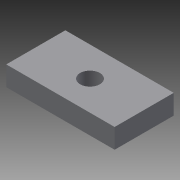
# Autodesk Inventor part: p1-1
Saved by Autodesk Inventor 2014 (Build 180170000, 170)
## iProperties
Created: 2017-02-06
Part Number: p1-1
Material: Generic
Document SubType Name: Modeling
Designer: mschaffel
Density: 1 g/cm^3
Appearance: Default
Author: mschaffel
Autodesk Inventor part; units mm, degrees
ref_plane "YZ Plane" through (0, 0, 0) normal (1, 0, 0) x (0, 1, 0)
ref_plane "XZ Plane" through (0, 0, 0) normal (0, 1, 0) x (-1, 0, 0)
ref_plane "XY Plane" through (0, 0, 0) normal (0, 0, 1) x (1, 0, 0)
sketch "Sketch1" plane through (0, 0, 0) normal (0, 1, 0) x (-1, 0, 0)
  line L0 (0, 0) -> (-139.7, 0)
  line L1 (-139.7, 0) -> (-139.7, 76.2)
  line L2 (-139.7, 76.2) -> (0, 76.2)
  line L3 (0, 76.2) -> (0, 0)
  dimension "d0" = 139.7
  dimension "d1" = 76.2
  constraints: 8 end point, 2 perpendicular, 1 horizontal, 1 parallel
  measures "d0" distance of L0.start L0.end
  measures "d1" distance of L0.end L1.end
extrude "Extrusion1" add sketch "Sketch1" along normal blind 25.4
sketch "Sketch2" plane through (0, 25.4, 0) normal (0, 1, 0) x (1, 0, 0)
  circle A0 centre (69.85, -38.1) radius 12.7
  dimension "d4" = 25.4
  constraints: 1 centre point
  measures "d4" diameter of A0
extrude "Extrusion2" cut sketch "Sketch2" against normal blind 25.4
body "Solid1"
